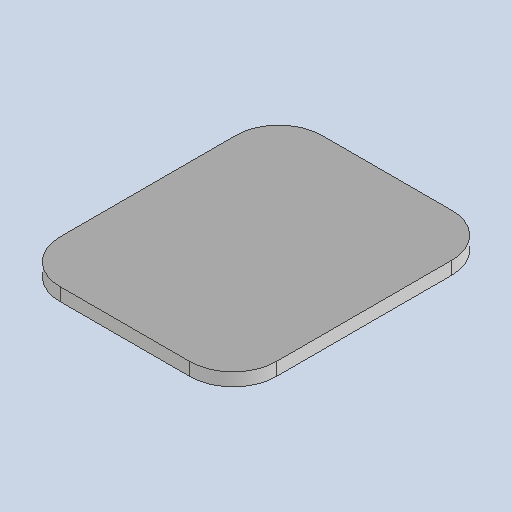
# Autodesk Inventor part: PRS 9694 leg plate for filter_D1200 940
Saved by Autodesk Inventor 2026.2 (Build 302298000, 298)
## iProperties
Created: 2025-02-20
Part Number: PRS 9694 leg plate for filter_D1200 940
Material: Stainless Steel
Document SubType Name: Sheet Metal
Designer: admin
Mass: 924.319 g
Surface Area: 416.673 cm^2
Volume: 115.54 cm^3
Density: 8 g/cm^3
Flat Pattern Width: 12.1198 cm
Flat Pattern Length: 10 cm
Flat Pattern Area: 121.198 cm^2
Sheet Metal Rule: AISI304 3mm Die 32
Sheet Metal Width: 121,198 mm
Sheet Metal Length: 100,000 mm
Sheet Metal Area: 12119,761 mm^2
Appearance: Default
Author: user
Autodesk Inventor part; units mm, degrees
ref_plane "YZ Plane" through (0, 0, 0) normal (1, 0, 0) x (0, 1, 0)
ref_plane "XZ Plane" through (0, 0, 0) normal (0, 1, 0) x (-1, 0, 0)
ref_plane "XY Plane" through (0, 0, 0) normal (0, 0, 1) x (1, 0, 0)
sketch "Sketch1" plane through (0, 0, 0) normal (0, 0, 1) x (1, 0, 0)
  line L0 (-50, -60.5988) -> (50, -60.5988)
  line L1 (50, -60.5988) -> (50, 60.5988)
  line L2 (50, 60.5988) -> (-50, 60.5988)
  line L3 (-50, 60.5988) -> (-50, -60.5988)
  line L4 (-50, -60.5988) -> (50, 60.5988) construction
  line L5 (50, -60.5988) -> (-50, 60.5988) construction
  point P0 (0, 0)
  dimension "d0" = 100
  dimension "d1" = 121.1976
  measures "d0" distance of L2.end L1.end
  measures "d1" distance of L1.end L0.end
extrude "Plate1" add sketch "Sketch1" along normal blind 6
fillet "Corner Round1" radius 20 4 edges at (50, -60.5988, 3) (-50, -60.5988, 3) (-50, 60.5988, 3) (50, 60.5988, 3)
sketch "Sketch5" plane through (0, 0, 6) normal (0, 0, 1) x (1, 0, 0)
  line L0 (50, 40.5988) -> (50, -40.5988) projected
  line L1 (50, 30.5988) -> (-50, 30.5988)
  line L2 (-50, -40.5988) -> (-50, 40.5988) projected
  line L3 (-30, 60.5988) -> (30, 60.5988) projected
  point P0 (0, 0)
  dimension "d23" = 30
  constraints: 2 end point, 2 point on line, 1 horizontal
  measures "d23" distance between parallel lines of L1 L3
feature "Fold1" [suppressed]
equation "\"d1\" = Legs_Upper_plate_lenght"
equation "\"d2\" = Thickness"
equation "\"d24\" = BendReliefWidth"
equation "\"d25\" = BendReliefDepth"
equation "\"d26\" = MinimumRemnant"
equation "\"d27\" = TransitionRadius"
equation "\"d29\" = BendRadius"
equation "\"BendReliefWidth\" = Thickness"
equation "\"BendReliefDepth\" = 0.5 * Thickness"
equation "\"CornerReliefSize\" = 4 * Thickness"
equation "\"MinimumRemnant\" = 2 * Thickness"
equation "\"TransitionRadius\" = BendRadius"
equation "\"JacobiRadiusSize\" = BendRadius"
equation "\"GapSize\" = Thickness"
equation "\"Legs_Upper_plate_lenght\" = 121.197614"
equation "\"Thickness\" = 6"
equation "\"BendRadius\" = 5"
body "Solid1"
